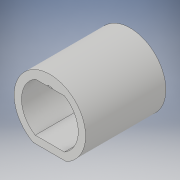
# Autodesk Inventor part: corridor
Saved by Autodesk Inventor 2017 (Build 210142000, 142)
## iProperties
Created: 2018-03-04
Part Number: corridor
Material: Generic
Document SubType Name: Modeling
Designer: Braxton
Density: 1 g/cm^3
Appearance: Default
Author: Braxton
Autodesk Inventor part; units mm, degrees
ref_plane "YZ Plane" through (0, 0, 0) normal (1, 0, 0) x (0, 1, 0)
ref_plane "XZ Plane" through (0, 0, 0) normal (0, 1, 0) x (-1, 0, 0)
ref_plane "XY Plane" through (0, 0, 0) normal (0, 0, 1) x (1, 0, 0)
sketch "Sketch1" plane through (0, 0, 0) normal (0, 0, 1) x (1, 0, 0)
  line L0 (-50.8, -84.6667) -> (50.8, -84.6667)
  arc A0 (57.793, -110.0667) -> (-57.793, -110.0667) centre (0, 0) ccw
  arc A1 (-50.8, 84.6667) -> (-50.8, -84.6667) centre (0, 0) ccw
  arc A2 (50.8, -84.6667) -> (50.8, 84.6667) centre (0, 0) ccw
  line L1 (-57.793, -110.0667) -> (57.793, -110.0667)
  line L2 (0, 84.6667) -> (0, 87.8417) construction
  line L3 (-7.4083, 87.8417) -> (7.4083, 87.8417)
  line L4 (-7.4083, 87.8417) -> (-7.4083, 86.2542)
  line L5 (7.4083, 87.8417) -> (7.4083, 86.2542)
  line L6 (8.9958, 84.6667) -> (50.8, 84.6667)
  line L7 (-8.9958, 84.6667) -> (8.9958, 84.6667) construction
  arc A3 (7.4083, 86.2542) -> (8.9958, 84.6667) centre (8.9958, 86.2542) ccw
  arc A4 (-8.9958, 84.6667) -> (-7.4083, 86.2542) centre (-8.9958, 86.2542) ccw
  line L8 (-8.9958, 84.6667) -> (-50.8, 84.6667)
  dimension "d1" = 101.6
  dimension "d20" = 25.4
  dimension "d21" = 124.3169
  dimension "d23" = 14.8167
  dimension "d27" = 98.7374
  dimension "d28" = 98.7374
  dimension "d30" = 43.3917
  dimension "d39" = 1.5875
  dimension "d40" = 1.5875
  dimension "d41" = 41.8042
  dimension "d44" = 3.175
  constraints: 18 end point, 11 point on circle, 5 centre point, 5 horizontal, 3 symmetric about line, 2 coincident, 2 perpendicular, 1 midpoint, 1 parallel, 1 tangent, 1 vertical, 1 other
  measures "d1" distance of L8.end L6.end
  measures "d20" distance between parallel lines of L0 L1
  measures "d21" radius of A0
  measures "d23" distance of L3.start L3.end
  measures "d27" radius of A1
  measures "d28" radius of A2
  measures "d30" distance from line of L8.end L4
  measures "d39" distance from line of L6.start L5
  measures "d40" radius of A3
  measures "d41" distance of L6.start L6.end
  measures "d44" distance from line of L3.end L6
extrude "corridor" add sketch "Sketch1" along normal blind 279.4
sketch "Sketch5" plane through (0, 0, 0) normal (0, 0, -1) x (-1, 0, 0)
  line L0 (-6.35, 87.8417) -> (0, 87.8417)
  line L1 (7.4083, 87.8417) -> (-7.4083, 87.8417) projected
  line L2 (-6.35, 87.8417) -> (-6.35, 86.6178)
  line L3 (-4.1034, 84.646) -> (0, 84.646)
  line L4 (0, 84.646) -> (0, 87.8417) construction
  line L5 (-6.3485, 84.6667) -> (-3.1743, 87.8409) construction
  arc A0 (-3.1736, 84.646) -> (-6.35, 87.8417) centre (-6.3485, 84.6667) ccw construction
  arc A1 (-6.35, 86.6178) -> (-4.1034, 84.646) centre (-4.1034, 86.9117) ccw
  line L6 (6.35, 87.8417) -> (0, 87.8417)
  line L7 (6.35, 87.8417) -> (6.35, 86.6178)
  line L8 (4.1034, 84.646) -> (0, 84.646)
  line L9 (6.3485, 84.6667) -> (3.1743, 87.8409) construction
  arc A2 (6.35, 87.8417) -> (3.1736, 84.646) centre (6.3485, 84.6667) ccw construction
  arc A3 (4.1034, 84.646) -> (6.35, 86.6178) centre (4.1034, 86.9117) ccw
  point P0 (0, 0)
  dimension "d31" = 6.35
  dimension "d32" = 3.175
  dimension "d34" = 45
  dimension "d35" = 2.2657
  dimension "d36" = 2.2466
  dimension "d45" = 1.2238
  constraints: 18 end point, 10 point on circle, 8 symmetric about line, 4 centre point, 4 point on line, 2 coincident, 2 perpendicular, 1 horizontal, 1 midpoint, 1 tangent, 1 vertical, 2 other
  measures "d31" distance of L0.end L0.start
  measures "d32" distance of L0.start L5.start
  measures "d34" angle of L0 L5
  measures "d35" radius of A1
  measures "d36" horizontal distance of L3.start L2.end
  measures "d45" distance of L6.start L7.end
extrude "light" add sketch "Sketch5" against normal up to surface (279.4 mm away) separate body
equation "\"d28\" = d27"
equation "\"d39\" = 0.5 * d26"
equation "\"d26\" = 3.175"
body "Solid1"
body "Solid2"
